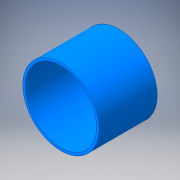
# Autodesk Inventor part: Part1
Saved by Autodesk Inventor 2016 (Build 200138000, 138)
## iProperties
Created: 2018-01-08
Part Number: Part1
Material: Generic
Document SubType Name: Modeling
Designer: sun01147
Density: 1 g/cm^3
Appearance: Default
Author: sun01147
Autodesk Inventor part; units mm, degrees
ref_plane "YZ Plane" through (0, 0, 0) normal (1, 0, 0) x (0, 1, 0)
ref_plane "XZ Plane" through (0, 0, 0) normal (0, 1, 0) x (-1, 0, 0)
ref_plane "XY Plane" through (0, 0, 0) normal (0, 0, 1) x (1, 0, 0)
sketch "Sketch1" plane through (0, 0, 0) normal (0, 0, 1) x (1, 0, 0)
  circle A0 centre (0, 0) radius 6.6749
  circle A1 centre (0, 0) radius 6.2226
  dimension "d0" = 13.3499
  dimension "d1" = 12.4451
  constraints: 2 centre point, 2 coincident
  measures "d0" diameter of A0
  measures "d1" diameter of A1
extrude "Extrusion1" add sketch "Sketch1" against normal blind 10.16
sketch "Sketch3" plane through (0, 0, -10.16) normal (0, 0, -1) x (-1, 0, 0)
  circle A0 centre (0, 0) radius 6.2226
  dimension "d6" = 12.4451
  constraints: 1 centre point, 1 coincident
  measures "d6" diameter of A0
extrude "Extrusion2" add sketch "Sketch3" against normal blind 0.635
body "Solid1"
